Autodesk Fusion 360 part; units mm, degrees
note: some values were not read from the file. Set by a fixed rule: which sketch regions a step uses.
(part 4 of 4)
sketch "Sketch64" plane through (0, 0, -20) normal (0, 0, -1) x (-1, 0, 0)
  line L0 (-150, -6) -> (150, -6)
  line L1 (150, -3) -> (-150, -3)
  line L2 (-150, 57) -> (150, 57)
  line L3 (150, 60) -> (-150, 60)
  line L4 (-150, 60) -> (-150, 57)
  line L5 (-150, -3) -> (-150, -6)
  line L6 (150, 57) -> (150, 60)
  line L7 (150, -6) -> (150, -3)
  line L8 (-152, 62) -> (-152, 55)
  line L9 (152, 55) -> (152, 62)
  line L10 (152, -8) -> (152, -1)
  line L11 (-152, -1) -> (-152, -8)
  line L12 (-129.3103, -16) -> (-139.6552, -16)
  line L13 (-139.6552, 70) -> (-129.3103, 70)
  line L14 (-139.6552, -1) -> (-152, -1)
  line L15 (-118.9655, -1) -> (-129.3103, -1)
  line L16 (-98.2759, -1) -> (-108.6207, -1)
  line L17 (-77.5862, -1) -> (-87.931, -1)
  line L18 (-56.8966, -1) -> (-67.2414, -1)
  line L19 (-36.2069, -1) -> (-46.5517, -1)
  line L20 (-15.5172, -1) -> (-25.8621, -1)
  line L21 (5.1724, -1) -> (-5.1724, -1)
  line L22 (25.8621, -1) -> (15.5172, -1)
  line L23 (46.5517, -1) -> (36.2069, -1)
  line L24 (67.2414, -1) -> (56.8966, -1)
  line L25 (87.931, -1) -> (77.5862, -1)
  line L26 (108.6207, -1) -> (98.2759, -1)
  line L27 (152, -1) -> (139.6552, -1)
  line L28 (129.3103, -1) -> (118.9655, -1)
  line L29 (-139.6552, -16) -> (-139.6552, -8)
  line L30 (-129.3103, -16) -> (-129.3103, -8)
  line L31 (-139.6552, -1) -> (-139.6552, 55)
  line L32 (-139.6552, 62) -> (-139.6552, 70)
  line L33 (-129.3103, -1) -> (-129.3103, 55)
  line L34 (-129.3103, 62) -> (-129.3103, 70)
  line L35 (-152, 55) -> (-139.6552, 55)
  line L36 (-139.6552, 62) -> (-152, 62)
  line L37 (-118.9655, -16) -> (-108.6207, -16)
  line L38 (-98.2759, -16) -> (-87.931, -16)
  line L39 (-77.5862, -16) -> (-67.2414, -16)
  line L40 (-56.8966, -16) -> (-46.5517, -16)
  line L41 (-36.2069, -16) -> (-25.8621, -16)
  line L42 (-15.5172, -16) -> (-5.1724, -16)
  line L43 (5.1724, -16) -> (15.5172, -16)
  line L44 (25.8621, -16) -> (36.2069, -16)
  line L45 (46.5517, -16) -> (56.8966, -16)
  line L46 (67.2414, -16) -> (77.5862, -16)
  line L47 (87.931, -16) -> (98.2759, -16)
  line L48 (108.6207, -16) -> (118.9655, -16)
  line L49 (129.3103, -16) -> (139.6552, -16)
  line L50 (-118.9655, 70) -> (-108.6207, 70)
  line L51 (-98.2759, 70) -> (-87.931, 70)
  line L52 (-77.5862, 70) -> (-67.2414, 70)
  line L53 (-56.8966, 70) -> (-46.5517, 70)
  line L54 (-36.2069, 70) -> (-25.8621, 70)
  line L55 (-15.5172, 70) -> (-5.1724, 70)
  line L56 (5.1724, 70) -> (15.5172, 70)
  line L57 (25.8621, 70) -> (36.2069, 70)
  line L58 (46.5517, 70) -> (56.8966, 70)
  line L59 (67.2414, 70) -> (77.5862, 70)
  line L60 (87.931, 70) -> (98.2759, 70)
  line L61 (108.6207, 70) -> (118.9655, 70)
  line L62 (129.3103, 70) -> (139.6552, 70)
  line L63 (-118.9655, -16) -> (-118.9655, -8)
  line L64 (-108.6207, -16) -> (-108.6207, -8)
  line L65 (-152, -8) -> (-139.6552, -8)
  line L66 (-129.3103, -8) -> (-118.9655, -8)
  line L67 (-108.6207, -8) -> (-98.2759, -8)
  line L68 (-87.931, -8) -> (-77.5862, -8)
  line L69 (-67.2414, -8) -> (-56.8966, -8)
  line L70 (-46.5517, -8) -> (-36.2069, -8)
  line L71 (-25.8621, -8) -> (-15.5172, -8)
  line L72 (-5.1724, -8) -> (5.1724, -8)
  line L73 (15.5172, -8) -> (25.8621, -8)
  line L74 (36.2069, -8) -> (46.5517, -8)
  line L75 (56.8966, -8) -> (67.2414, -8)
  line L76 (77.5862, -8) -> (87.931, -8)
  line L77 (98.2759, -8) -> (108.6207, -8)
  line L78 (118.9655, -8) -> (129.3103, -8)
  line L79 (139.6552, -8) -> (152, -8)
  line L80 (-98.2759, -16) -> (-98.2759, -8)
  line L81 (-87.931, -16) -> (-87.931, -8)
  line L82 (-77.5862, -16) -> (-77.5862, -8)
  line L83 (-67.2414, -16) -> (-67.2414, -8)
  line L84 (-56.8966, -16) -> (-56.8966, -8)
  line L85 (-46.5517, -16) -> (-46.5517, -8)
  line L86 (-36.2069, -16) -> (-36.2069, -8)
  line L87 (-25.8621, -16) -> (-25.8621, -8)
  line L88 (-15.5172, -16) -> (-15.5172, -8)
  line L89 (-5.1724, -16) -> (-5.1724, -8)
  line L90 (5.1724, -16) -> (5.1724, -8)
  line L91 (15.5172, -16) -> (15.5172, -8)
  line L92 (25.8621, -16) -> (25.8621, -8)
  line L93 (36.2069, -16) -> (36.2069, -8)
  line L94 (46.5517, -16) -> (46.5517, -8)
  line L95 (56.8966, -16) -> (56.8966, -8)
  line L96 (67.2414, -16) -> (67.2414, -8)
  line L97 (77.5862, -16) -> (77.5862, -8)
  line L98 (87.931, -16) -> (87.931, -8)
  line L99 (98.2759, -16) -> (98.2759, -8)
  line L100 (108.6207, -16) -> (108.6207, -8)
  line L101 (118.9655, -16) -> (118.9655, -8)
  line L102 (129.3103, -16) -> (129.3103, -8)
  line L103 (139.6552, -16) -> (139.6552, -8)
  line L104 (-118.9655, -1) -> (-118.9655, 55)
  line L105 (-118.9655, 62) -> (-118.9655, 70)
  line L106 (-118.9655, 62) -> (-129.3103, 62)
  line L107 (-108.6207, -1) -> (-108.6207, 55)
  line L108 (-108.6207, 62) -> (-108.6207, 70)
  line L109 (-129.3103, 55) -> (-118.9655, 55)
  line L110 (-98.2759, -1) -> (-98.2759, 55)
  line L111 (-98.2759, 62) -> (-98.2759, 70)
  line L112 (-108.6207, 55) -> (-98.2759, 55)
  line L113 (-98.2759, 62) -> (-108.6207, 62)
  line L114 (-87.931, -1) -> (-87.931, 55)
  line L115 (-87.931, 62) -> (-87.931, 70)
  line L116 (-77.5862, -1) -> (-77.5862, 55)
  line L117 (-77.5862, 62) -> (-77.5862, 70)
  line L118 (-87.931, 55) -> (-77.5862, 55)
  line L119 (-77.5862, 62) -> (-87.931, 62)
  line L120 (-67.2414, -1) -> (-67.2414, 55)
  line L121 (-67.2414, 62) -> (-67.2414, 70)
  line L122 (-67.2414, 55) -> (-56.8966, 55)
  line L123 (-56.8966, 62) -> (-67.2414, 62)
  line L124 (-56.8966, -1) -> (-56.8966, 55)
  line L125 (-56.8966, 62) -> (-56.8966, 70)
  line L126 (-46.5517, -1) -> (-46.5517, 55)
  line L127 (-46.5517, 62) -> (-46.5517, 70)
  line L128 (-36.2069, -1) -> (-36.2069, 55)
  line L129 (-36.2069, 62) -> (-36.2069, 70)
  line L130 (-36.2069, 62) -> (-46.5517, 62)
  line L131 (-46.5517, 55) -> (-36.2069, 55)
  line L132 (-25.8621, -1) -> (-25.8621, 55)
  line L133 (-25.8621, 62) -> (-25.8621, 70)
  line L134 (-25.8621, 55) -> (-15.5172, 55)
  line L135 (-15.5172, 62) -> (-25.8621, 62)
  line L136 (-15.5172, -1) -> (-15.5172, 55)
  line L137 (-15.5172, 62) -> (-15.5172, 70)
  line L138 (-5.1724, -1) -> (-5.1724, 55)
  line L139 (-5.1724, 62) -> (-5.1724, 70)
  line L140 (-5.1724, 55) -> (5.1724, 55)
  line L141 (5.1724, 62) -> (-5.1724, 62)
  line L142 (5.1724, -1) -> (5.1724, 55)
  line L143 (5.1724, 62) -> (5.1724, 70)
  line L144 (15.5172, -1) -> (15.5172, 55)
  line L145 (15.5172, 62) -> (15.5172, 70)
  line L146 (15.5172, 55) -> (25.8621, 55)
  line L147 (25.8621, 62) -> (15.5172, 62)
  line L148 (25.8621, -1) -> (25.8621, 55)
  line L149 (25.8621, 62) -> (25.8621, 70)
  line L150 (36.2069, -1) -> (36.2069, 55)
  line L151 (36.2069, 62) -> (36.2069, 70)
  line L152 (36.2069, 55) -> (46.5517, 55)
  line L153 (46.5517, -1) -> (46.5517, 55)
  line L154 (46.5517, 62) -> (46.5517, 70)
  line L155 (46.5517, 62) -> (36.2069, 62)
  line L156 (56.8966, -1) -> (56.8966, 55)
  line L157 (56.8966, 62) -> (56.8966, 70)
  line L158 (67.2414, -1) -> (67.2414, 55)
  line L159 (67.2414, 62) -> (67.2414, 70)
  line L160 (67.2414, 62) -> (56.8966, 62)
  line L161 (56.8966, 55) -> (67.2414, 55)
  line L162 (77.5862, -1) -> (77.5862, 55)
  line L163 (77.5862, 62) -> (77.5862, 70)
  line L164 (77.5862, 55) -> (87.931, 55)
  line L165 (87.931, 62) -> (77.5862, 62)
  line L166 (87.931, -1) -> (87.931, 55)
  line L167 (87.931, 62) -> (87.931, 70)
  line L168 (98.2759, -1) -> (98.2759, 55)
  line L169 (98.2759, 62) -> (98.2759, 70)
  line L170 (108.6207, -1) -> (108.6207, 55)
  line L171 (108.6207, 62) -> (108.6207, 70)
  line L172 (108.6207, 62) -> (98.2759, 62)
  line L173 (118.9655, -1) -> (118.9655, 55)
  line L174 (118.9655, 62) -> (118.9655, 70)
  line L175 (98.2759, 55) -> (108.6207, 55)
  line L176 (129.3103, -1) -> (129.3103, 55)
  line L177 (129.3103, 62) -> (129.3103, 70)
  line L178 (118.9655, 55) -> (129.3103, 55)
  line L179 (139.6552, 55) -> (152, 55)
  line L180 (152, 62) -> (139.6552, 62)
  line L181 (129.3103, 62) -> (118.9655, 62)
  line L182 (139.6552, -1) -> (139.6552, 55)
  line L183 (139.6552, 62) -> (139.6552, 70)
  point P0 (150, -16)
  point P1 (150, 70)
  dimension "d743" = 10
  constraint coincident L15.end L30
  constraint coincident L14.start L29
  constraint collinear L14 L27
  constraint coincident L16.end L64
  constraint coincident L15.start L63
  constraint collinear L15 L27
  constraint coincident L17.end L81
  constraint coincident L16.start L80
  constraint collinear L16 L27
  constraint coincident L18.end L83
  constraint coincident L17.start L82
  constraint collinear L17 L27
  constraint coincident L19.end L85
  constraint coincident L18.start L84
  constraint collinear L18 L27
  constraint coincident L20.end L87
  constraint coincident L19.start L86
  constraint collinear L19 L27
  constraint coincident L21.end L89
  constraint coincident L20.start L88
  constraint collinear L20 L27
  constraint coincident L22.end L91
  constraint coincident L21.start L90
  constraint collinear L21 L27
  constraint coincident L23.end L93
  constraint coincident L22.start L92
  constraint collinear L22 L27
  constraint coincident L24.end L95
  constraint coincident L23.start L94
  constraint collinear L23 L27
  constraint coincident L25.end L97
  constraint coincident L24.start L96
  constraint collinear L24 L27
  constraint coincident L26.end L99
  constraint coincident L25.start L98
  constraint collinear L25 L27
  constraint coincident L28.end L101
  constraint coincident L26.start L100
  constraint collinear L26 L27
  constraint coincident L27.end L103
  constraint coincident L28.start L102
  constraint collinear L27 L28
  constraint collinear L29 L31
  constraint collinear L30 L33
  constraint coincident L30.end L65
  constraint collinear L31 L32
  constraint coincident L32.start L180
  constraint collinear L33 L34
  constraint coincident L33.end L35
  constraint collinear L35 L109
  constraint collinear L36 L180
  constraint perpendicular L37 L64
  constraint perpendicular L38 L81
  constraint perpendicular L39 L83
  constraint perpendicular L40 L85
  constraint perpendicular L41 L87
  constraint perpendicular L42 L89
  constraint perpendicular L43 L91
  constraint perpendicular L44 L93
  constraint perpendicular L45 L95
  constraint perpendicular L46 L97
  constraint perpendicular L47 L99
  constraint perpendicular L48 L101
  constraint perpendicular L49 L103
  constraint perpendicular L50 L64
  constraint perpendicular L51 L81
  constraint perpendicular L52 L83
  constraint perpendicular L53 L84
  constraint perpendicular L54 L87
  constraint perpendicular L55 L89
  constraint perpendicular L56 L91
  constraint perpendicular L57 L93
  constraint perpendicular L58 L95
  constraint perpendicular L59 L97
  constraint perpendicular L60 L99
  constraint perpendicular L61 L101
  constraint perpendicular L62 L102
  constraint collinear L63 L104
  constraint collinear L64 L107
  constraint coincident L64.end L65
  constraint collinear L65 L67
  constraint collinear L65 L66
  constraint collinear L67 L68
  constraint collinear L68 L69
  constraint collinear L69 L70
  constraint collinear L70 L71
  constraint collinear L71 L72
  constraint collinear L72 L73
  constraint collinear L73 L74
  constraint collinear L74 L75
  constraint collinear L75 L76
  constraint collinear L76 L77
  constraint collinear L77 L78
  constraint collinear L78 L79
  constraint collinear L80 L110
  constraint collinear L81 L114
  constraint collinear L84 L124
  constraint collinear L86 L128
  constraint collinear L88 L136
  constraint collinear L89 L138
  constraint collinear L90 L142
  constraint collinear L92 L148
  constraint collinear L94 L153
  constraint collinear L95 L156
  constraint collinear L97 L162
  constraint collinear L99 L168
  constraint collinear L101 L173
  constraint collinear L103 L182
  constraint collinear L104 L105
  constraint coincident L105.start L180
  constraint coincident L108.start L107
  constraint collinear L106 L180
  constraint collinear L107 L108
  constraint coincident L107.end L109
  constraint collinear L109 L112
  constraint collinear L110 L111
  constraint collinear L112 L118
  constraint coincident L111.start L180
  constraint coincident L115.start L114
  constraint collinear L113 L180
  constraint collinear L114 L115
  constraint collinear L116 L117
  constraint collinear L118 L122
  constraint coincident L117.start L180
  constraint coincident L121.start L120
  constraint collinear L119 L180
  constraint collinear L120 L121
  constraint collinear L122 L131
  constraint coincident L127.start L126
  constraint coincident L123.start L124
  constraint collinear L123 L180
  constraint collinear L124 L125
  constraint collinear L126 L127
  constraint collinear L128 L129
  constraint coincident L129.start L180
  constraint coincident L133.start L132
  constraint collinear L130 L180
  constraint collinear L131 L134
  constraint collinear L132 L133
  constraint collinear L134 L140
  constraint coincident L139.start L138
  constraint coincident L135.start L136
  constraint collinear L135 L180
  constraint collinear L136 L137
  constraint collinear L138 L139
  constraint collinear L140 L146
  constraint coincident L145.start L144
  constraint coincident L141.start L142
  constraint collinear L141 L180
  constraint collinear L142 L143
  constraint collinear L144 L145
  constraint collinear L146 L152
  constraint coincident L151.start L150
  constraint coincident L147.start L148
  constraint collinear L147 L180
  constraint collinear L148 L149
  constraint collinear L150 L151
  constraint collinear L152 L161
  constraint collinear L153 L154
  constraint coincident L154.start L180
  constraint coincident L157.start L156
  constraint collinear L155 L180
  constraint collinear L156 L157
  constraint collinear L158 L159
  constraint coincident L159.start L180
  constraint coincident L163.start L162
  constraint collinear L160 L180
  constraint collinear L161 L164
  constraint collinear L162 L163
  constraint collinear L164 L175
  constraint coincident L169.start L168
  constraint coincident L165.start L166
  constraint collinear L165 L180
  constraint collinear L166 L167
  constraint collinear L168 L169
  constraint collinear L170 L171
  constraint coincident L171.start L180
  constraint coincident L174.start L173
  constraint collinear L172 L180
  constraint collinear L173 L174
  constraint coincident L173.end L175
  constraint collinear L175 L178
  constraint collinear L176 L177
  constraint collinear L178 L179
  constraint coincident L177.start L180
  constraint coincident L180.end L182
  constraint collinear L180 L181
  constraint collinear L182 L183
  measures "d743" distance of L0.end P0
extrude "Extrude98" add sketch "Sketch64" against normal blind 3 separate body makes body 98
